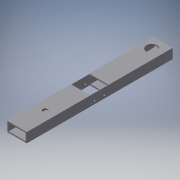
# Autodesk Inventor part: 1x2 arm
Saved by Autodesk Inventor 2018 (Build 220112000, 112)
## iProperties
Created: 2018-01-20
Part Number: 1x2 arm
Material: Generic
Document SubType Name: Modeling
Designer: Apple
Density: 1 g/cm^3
Appearance: Default
Author: Apple
Autodesk Inventor part; units mm, degrees
ref_plane "YZ Plane" through (0, 0, 0) normal (1, 0, 0) x (0, 1, 0)
ref_plane "XZ Plane" through (0, 0, 0) normal (0, 1, 0) x (-1, 0, 0)
ref_plane "XY Plane" through (0, 0, 0) normal (0, 0, 1) x (1, 0, 0)
sketch "Sketch1" plane through (0, 0, 0) normal (0, 0, 1) x (1, 0, 0)
  line L0 (-59.9006, 6.3636) -> (-15.4506, 6.3636)
  line L1 (-15.4506, 6.3636) -> (-15.4506, -12.6864)
  line L2 (-15.4506, -12.6864) -> (-59.9006, -12.6864)
  line L3 (-59.9006, -12.6864) -> (-59.9006, 6.3636)
  line L4 (-63.0756, 9.5386) -> (-12.2756, 9.5386)
  line L5 (-12.2756, 9.5386) -> (-12.2756, -15.8614)
  line L6 (-12.2756, -15.8614) -> (-63.0756, -15.8614)
  line L7 (-63.0756, -15.8614) -> (-63.0756, 9.5386)
  point P0 (0, 0)
  dimension "d2" = 3.175
  dimension "d5" = 50.8
  dimension "d6" = 25.4
  constraints: 16 end point, 4 parallel, 2 perpendicular, 1 horizontal, 3 other
  measures "d2" distance between parallel lines of L3 L7
  measures "d5" distance between parallel lines of L5 L7
  measures "d6" distance of L6.end L4.start
extrude "Extrusion1" add sketch "Sketch1" along normal blind 381
sketch "Sketch4" plane through (-63.0756, 9.5386, 0) normal (0, 1, 0) x (1, 0, 0)
  circle A0 centre (24.9171, -28.575) radius 14.2621
  line L0 (0, 0) -> (50.8, 0) projected
  point P0 (63.0756, 0)
  dimension "d13" = 28.5242
  dimension "d14" = 28.575
  constraints: 1 centre point
  measures "d13" diameter of A0
  measures "d14" distance from line of L0 A0.centre
extrude "Extrusion4" cut sketch "Sketch4" against normal through all
sketch "Sketch2" plane through (-63.0756, 9.5386, 0) normal (0, 1, 0) x (1, 0, 0)
  line L0 (1.5875, -167.2625) -> (49.2125, -167.2625)
  line L1 (49.2125, -167.2625) -> (49.2125, -214.8875)
  line L2 (49.2125, -214.8875) -> (1.5875, -214.8875)
  line L3 (1.5875, -214.8875) -> (1.5875, -167.2625)
  line L4 (50.8, -381) -> (0, -381) projected
  circle A0 centre (24.9171, -28.575) radius 14.2621 projected
  point P0 (63.0756, 0)
  point P1 (25.4, -214.8875)
  point P2 (25.4, -381)
  dimension "d7" = 47.625
  dimension "d8" = 47.625
  dimension "d17" = 138.6875
  constraints: 8 end point, 2 midpoint, 2 parallel, 1 horizontal, 1 perpendicular, 1 vertical alignment
  measures "d7" distance of L0.start L0.end
  measures "d8" distance of L0.end L1.end
  measures "d17" distance from line of L0 A0.centre
extrude "Extrusion2" cut sketch "Sketch2" against normal through all contours L0 L1 L2 L3
sketch "Sketch5" plane through (-12.2756, -15.8614, 0) normal (1, 0, 0) x (0, 0, -1)
  circle A0 centre (-203.775, 7.5085) radius 2.0193 projected
  circle A1 centre (-178.375, 7.5085) radius 2.0193 projected
  point P0 (0, 15.8614)
extrude "Extrusion5" cut sketch "Sketch5" against normal through all
sketch "Sketch6" plane through (-63.0756, -15.8614, 0) normal (0, -1, 0) x (1, 0, 0)
  circle A0 centre (25.4, 307.975) radius 6.35 projected
  point P0 (63.0756, 0)
extrude "Extrusion6" cut sketch "Sketch6" against normal through all
equation "\"d8\" = d7"
body "Solid1"
